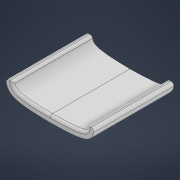
# Autodesk Inventor part: SeatBase
Saved by Autodesk Inventor 2021 (Build 250183000, 183)
## iProperties
Created: 2021-01-30
Part Number: SeatBase
Material: Generic
Document SubType Name: Modeling
Designer: argon
Density: 1 g/cm^3
Appearance: Default
Author: argon
Autodesk Inventor part; units mm, degrees
ref_plane "YZ Plane" through (0, 0, 0) normal (1, 0, 0) x (0, 1, 0)
ref_plane "XZ Plane" through (0, 0, 0) normal (0, 1, 0) x (-1, 0, 0)
ref_plane "XY Plane" through (0, 0, 0) normal (0, 0, 1) x (1, 0, 0)
sketch "Sketch1" plane through (0, 0, 0) normal (0, 0, 1) x (1, 0, 0)
  line L0 (0, 0) -> (-187.4869, 3.2416) construction
  line L1 (-187.4869, 3.2416) -> (-234.6064, 12.8161) construction
  line L2 (-234.6064, 12.8161) -> (-275, 37.6892) construction
  line L3 (-275, 37.6892) -> (-275, 101.7619) construction
  spline S0 degree 4 poles (0, 0) (-187.4869, 3.2416) (-234.6064, 12.8161) (-275, 37.6892) (-275, 101.7619) knots 1 1 1 1 1 2 2 2 2 2
  line L4 (0, 0) -> (0, 113.2924) construction
  line L5 (0, 0) -> (187.4869, 3.2416) construction
  line L6 (187.4869, 3.2416) -> (234.6064, 12.8161) construction
  line L7 (234.6064, 12.8161) -> (275, 37.6892) construction
  line L8 (275, 37.6892) -> (275, 101.7619) construction
  spline S1 degree 4 poles (0, 0) (187.4869, 3.2416) (234.6064, 12.8161) (275, 37.6892) (275, 101.7619) knots 1 1 1 1 1 2 2 2 2 2
  line L9 (-275, 101.7619) -> (-235, 101.7619)
  line L10 (275, 101.7619) -> (235, 101.7619)
  spline S2 degree 5 poles (-235, 101.7619) (-234.9998, 98.1416) (-234.829, 94.5189) (-234.4531, 90.9128) (-233.4432, 85.0816) (-231.5323, 79.4999) (-230.6428, 77.4013) (-228.5783, 73.5846) (-225.8087, 70.2481) (-224.3404, 68.804) (-220.2503, 65.3804) (-215.6211, 62.6959) (-212.6781, 61.2498) (-204.6005, 57.7948) (-196.1783, 55.2591) (-190.846, 53.8937) (-177.3264, 50.9118) (-163.6377, 48.8133) (-155.3667, 47.7495) (-135.3378, 45.5582) (-115.2425, 44.075) (-103.4552, 43.3581) (-75.702, 41.9491) (-47.9275, 41.0412) (-31.9532, 40.623) (-15.9771, 40.2844) (0, 40.006) knots 0 0 0 0 0 0 0.068525 0.068525 0.068525 0.111462 0.111462 0.111462 0.150213 0.150213 0.150213 0.212189 0.212189 0.212189 0.316307 0.316307 0.316307 0.474099 0.474099 0.474099 0.697579 0.697579 0.697579 1 1 1 1 1 1
  spline S3 degree 5 poles (0, 40.006) (15.9771, 40.2844) (31.9532, 40.623) (47.9275, 41.0412) (75.702, 41.9491) (103.4552, 43.3581) (115.2425, 44.075) (135.3378, 45.5582) (155.3667, 47.7495) (163.6377, 48.8133) (177.3264, 50.9118) (190.846, 53.8937) (196.1783, 55.2591) (204.6005, 57.7948) (212.6781, 61.2498) (215.6211, 62.6959) (220.2503, 65.3804) (224.3404, 68.804) (225.8087, 70.2481) (228.5783, 73.5846) (230.6428, 77.4013) (231.5323, 79.4999) (233.4432, 85.0816) (234.4531, 90.9128) (234.829, 94.5189) (234.9998, 98.1416) (235, 101.7619) knots 0 0 0 0 0 0 0.302421 0.302421 0.302421 0.525901 0.525901 0.525901 0.683693 0.683693 0.683693 0.787811 0.787811 0.787811 0.849787 0.849787 0.849787 0.888538 0.888538 0.888538 0.931475 0.931475 0.931475 1 1 1 1 1 1
  dimension "d3" = 40
  dimension "d0" = 275
  constraints: 6 end point, 4 symmetric about line, 2 vertical, 1 collinear, 1 horizontal, 12 other
  measures "d0" horizontal distance of L3.end L0.start
extrude "Extrusion1" add sketch "Sketch1" along normal blind 500
fillet "Fillet1" radius 16 6 edges at (-275, 101.7619, 250) (-235, 101.7619, 250) (235, 101.7619, 250) (275, 101.7619, 250) (-131.9618, 45.4436, 500) (131.9618, 45.4436, 500)
body "Solid1"
